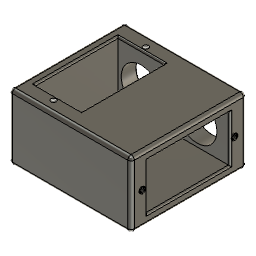
Hinge00 (Autodesk Fusion 360 design; units mm, degrees)
part number: 2026-06-04-09-57-52-596
Autodesk Fusion 360 part; units mm, degrees
sketch "Sketch1" plane through (0, 0, 0) normal (0, 0, 1) x (1, 0, 0)
  line L0 (18.5, -17.5) -> (-18.5, -17.5)
  line L1 (-18.5, -17.5) -> (-18.5, 17.5)
  line L2 (-18.5, 17.5) -> (18.5, 17.5)
  line L3 (18.5, 17.5) -> (18.5, -17.5)
  line L4 (18.5, -17.5) -> (-18.5, 17.5) construction
  line L5 (-18.5, -17.5) -> (18.5, 17.5) construction
  dimension "d1" = 35
  dimension "d2" = 37
  constraint horizontal L0
  constraint perpendicular L0 L1
  constraint parallel L0 L2
  constraint parallel L1 L3
  constraint coincident L4 origin
  constraint coincident L5 origin
  measures "d1" distance of L0.end L1.end
  measures "d2" distance of L1.end L2.end
extrude "Extrude1" add sketch "Sketch1" along normal blind 20
sketch "Sketch4" plane through (18.5, 0, 0) normal (1, 0, 0) x (0, 1, 0)
  line L0 (-17.5, 0) -> (17.5, 0)
  line L1 (17.5, 0) -> (17.5, 20)
  line L2 (17.5, 20) -> (-17.5, 20)
  line L3 (-17.5, 20) -> (-17.5, 0)
  line L4 (12.5, 3) -> (-12.5, 3)
  line L5 (-12.5, 3) -> (-12.5, 17)
  line L6 (-12.5, 17) -> (12.5, 17)
  line L7 (12.5, 17) -> (12.5, 3)
  line L8 (12.5, 3) -> (-12.5, 17) construction
  line L9 (-12.5, 3) -> (12.5, 17) construction
  point P0 (0, 10)
  dimension "d39" = 25
  dimension "d40" = 14
  dimension "d41" = 10
  constraint horizontal L4
  constraint perpendicular L4 L5
  constraint parallel L4 L6
  constraint parallel L5 L7
  constraint coincident L8 P0
  constraint coincident L9 P0
  measures "d39" distance of L5.end L6.end
  measures "d40" distance of L4.end L5.end
  measures "d41" distance of origin P0
extrude "Extrude3" cut sketch "Sketch4" against normal blind 17 contours L4 L5 L6 L7
sketch "Sketch5" plane through (18.5, 0, 0) normal (1, 0, 0) x (0, 1, 0)
  line L0 (-12.5, 3) -> (-12.5, 17)
  line L1 (-12.5, 17) -> (12.5, 17)
  line L2 (12.5, 17) -> (12.5, 3)
  line L3 (12.5, 3) -> (-12.5, 3)
  line L4 (-17.5, 0) -> (17.5, 0)
  line L5 (17.5, 0) -> (17.5, 20)
  line L6 (17.5, 20) -> (-17.5, 20)
  line L7 (-17.5, 20) -> (-17.5, 0)
  point P0 (-14, 10)
  point P1 (14, 10)
  dimension "d44" = 1.5
  dimension "d45" = 1.5
  dimension "d46" = 10
  dimension "d47" = 10
  measures "d44" distance of L0 P0
  measures "d45" distance of L2 P1
  measures "d46" distance of L4 P1
  measures "d47" distance of L4 P0
hole "Hole3" at (18.5, -14, 10) at (18.5, 14, 10) direction (-1, 0, 0) diameter 1.623 depth 6 tip angle 118
thread "Thread2" "ISO Metric profile 2.0 M2x0.4 M2x0.4 6H" major diameter 2.074 minor diameter 1.623 pitch 0.4 angle 60 modelled right hand crest width 0.1065 on face at (14.5, 14.0808, 9.1925) crest through (18.4, 14.8115, 10) on face at (14.5, -13.9192, 9.1925) crest through (18.4, -13.1885, 10)
hole "Hole4" at (8.5, 17.5, 10) direction (0, -1, 0) diameter 12 depth 5 tip angle 180
sketch "Sketch6" plane through (0, 0, 20) normal (0, 0, 1) x (-1, 0, 0)
  line L0 (-18.5, -17.5) -> (18.5, -17.5)
  line L1 (18.5, -17.5) -> (18.5, 17.5)
  line L2 (18.5, 17.5) -> (-18.5, 17.5)
  line L3 (-18.5, 17.5) -> (-18.5, -17.5)
  line L4 (15.5, -12.5) -> (1.5, -12.5)
  line L5 (1.5, -12.5) -> (1.5, 12.5)
  line L6 (1.5, 12.5) -> (15.5, 12.5)
  line L7 (15.5, 12.5) -> (15.5, -12.5)
  point P0 (15.5, 0)
  dimension "d58" = 14
  dimension "d59" = 25
  dimension "d60" = 20
  dimension "d61" = 17.5
  constraint horizontal L4
  constraint vertical L5
  constraint horizontal L6
  constraint vertical L7
  constraint coincident L7 P0
  constraint midpoint L7 P0
  measures "d58" distance of L4.start L4.end
  measures "d59" distance of L4.start L6.end
  measures "d60" distance of L3 L5
  measures "d61" distance of L0 P0
extrude "Extrude4" cut sketch "Sketch6" against normal blind 17 contours L4 L5 L6 L7
sketch "Sketch7" plane through (0, 0, 20) normal (0, 0, 1) x (-1, 0, 0)
  line L0 (1.5, -12.5) -> (1.5, 12.5)
  line L1 (1.5, 12.5) -> (15.5, 12.5)
  line L2 (15.5, 12.5) -> (15.5, -12.5)
  line L3 (15.5, -12.5) -> (1.5, -12.5)
  line L4 (-18.5, -17.5) -> (18.5, -17.5)
  line L5 (18.5, -17.5) -> (18.5, 17.5)
  line L6 (18.5, 17.5) -> (-18.5, 17.5)
  line L7 (-18.5, 17.5) -> (-18.5, -17.5)
  point P0 (8.5, 14)
  point P1 (8.5, -14)
  dimension "d64" = 1.5
  dimension "d65" = 1.5
  dimension "d66" = 7
  dimension "d67" = 7
  measures "d64" distance of L3 P1
  measures "d65" distance of L1 P0
  measures "d66" horizontal distance of L2.end P1
  measures "d67" horizontal distance of L0.end P0
hole "Hole5" at (-8.5, -14, 20) at (-8.5, 14, 20) direction (0, 0, -1) diameter 1.623 depth 6 tip angle 118
thread "Thread3" "ISO Metric profile 2.0 M2x0.4 M2x0.4 6H" thread offset 0 thread depth 7.4
hole "Hole6" at (-8.5, 17.5, 10) direction (0, -1, 0) diameter 12 depth 5 tip angle 180
fillet "Fillet3" radius 0.5 10 edges at (18.5, -12.5, 10) (18.5, 0, 17) (18.5, 12.5, 10) (18.5, 0, 3) (10.6697, 17.5, 4.406) (-6.3303, 17.5, 4.406) (-1.5, 0, 20) (-8.5, 12.5, 20) (-15.5, 0, 20) (-8.5, -12.5, 20)
fillet "Fillet4" radius 1 12 edges at (-18.5, 0, 20) (0, -17.5, 20) (-18.5, -17.5, 10) (18.5, 0, 20) (0, 17.5, 20) (18.5, -17.5, 10) (0, -17.5, 0) (-18.5, 0, 0) (-18.5, 17.5, 10) (0, 17.5, 0) (18.5, 17.5, 10) (18.5, 0, 0)
